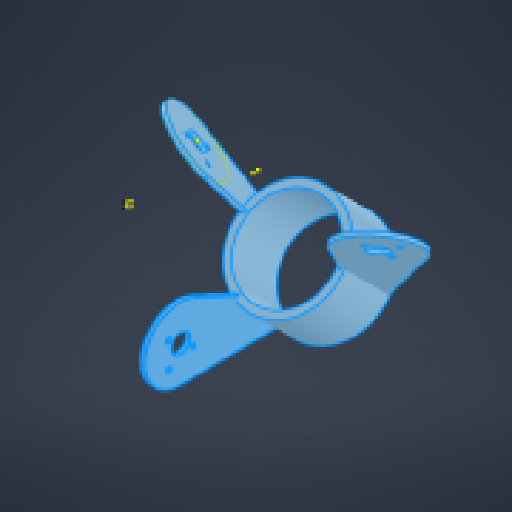
# Autodesk Inventor part: Base3MotorsHead
Saved by Autodesk Inventor 2026 (Build 300175050, 175E)
## iProperties
Created: 2025-06-26
Part Number: Base3MotorsHead
Material: Generic
Document SubType Name: Modeling
Designer: RubenPC
Density: 1 g/cm^3
Appearance: Default
Author: RubenPC
Autodesk Inventor part; units mm, degrees
ref_plane "Work Plane2" through (-10.193577, 19.428351, 24.333337) normal (0.5, 0.6123724, -0.6123724) x (-0.8659961, 0.3593609, -0.3477219)
sketch "Sketch1" plane through (-10.193577, 19.428351, 24.333337) normal (0.5, 0.6123724, -0.6123724) x (-0.8659961, 0.3593609, -0.3477219)
  circle A0 centre (-11.136116, 17.567445) radius 13.35
  circle A1 centre (-11.136116, 9.567445) radius 1.3
  circle A2 centre (-11.136116, 25.567445) radius 1.3
  circle A3 centre (-22.136116, 17.567445) radius 1.3
  circle A4 centre (-11.136116, 17.567445) radius 5
  circle A5 centre (-11.136116, 17.567445) radius 19.05
  point P0 (-7.348153, -30.884757)
  dimension "d3" = 38.1
  constraints: 1 centre point, 1 coincident
  measures "d3" diameter of A5
extrude "Extrusion1" add sketch "Sketch1" along normal blind 2 contours A0 | A5
ref_plane "Work Plane3" through (38.369556, -40.049097, 83.810785) normal (1, 0, 0) x (0, 0.8165027, -0.5773415)
ref_plane "Work Plane4" through (38.369556, -40.049097, 83.810785) normal (1, 0, 0) x (0, 0.8165027, -0.5773415)
sketch "Sketch2" plane through (38.369556, -40.049097, 83.810785) normal (1, 0, 0) x (0, 0.8165027, -0.5773415)
  circle A0 centre (14.07312, 15.315857) radius 13.35
  circle A1 centre (14.07312, 7.315857) radius 1.3
  circle A2 centre (14.07312, 23.315857) radius 1.3
  circle A3 centre (3.07312, 15.315857) radius 1.3
  circle A4 centre (14.07312, 15.315857) radius 5
  circle A5 centre (14.07312, 15.315857) radius 19.05
  point P0 (81.087646, -45.309729)
  dimension "d2" = 38.1
  constraints: 1 centre point, 1 coincident
  measures "d2" diameter of A5
extrude "Extrusion2" add sketch "Sketch2" along normal blind 2 separate body contours A0 | A5
ref_plane "Work Plane5" through (77.39899, 56.579392, 52.285482) normal (0.5, -0.6123724, 0.6123724) x (0.7923994, 0.6088063, -0.038185)
sketch "Sketch4" plane through (0.575465, 29.021734, 39.45362) normal (0.5, 0.6123724, -0.6123724) x (-0.7745967, 0, -0.6324555)
  circle A0 centre (0, 0) radius 19.05 projected
  circle A1 centre (0, 0) radius 19.05 projected
  point P0 (25.398414, -41.435313)
sketch "Sketch8" plane through (-10.193577, 19.428351, 24.333337) normal (0.5, 0.6123724, -0.6123724) x (-0.8659961, 0.3593609, -0.3477219)
  circle A0 centre (-11.136116, 17.567445) radius 19.05
  line L0 (-29.456151, 22.790356) -> (-37.949033, 0.312331)
  line L1 (-38.236466, -34.611486) -> (2.996032, 4.79306)
  line L2 (-38.236466, -34.611486) -> (-37.949033, 0.312331)
  point P0 (-7.348153, -30.884757)
  point P1 (0.984757, 2.87095)
  point P2 (-30.144601, 16.31047)
  constraints: 6 end point, 2 point on circle, 3 other
ref_plane "Work Plane7" through (48.769556, 20.910804, 22.850885) normal (0, 0.7071068, 0.7071068) x (0, 0.7071068, -0.7071068)
sketch "Sketch11" plane through (48.769556, 20.910804, 22.850885) normal (0, 0.7071068, 0.7071068) x (0, 0.7071068, -0.7071068)
  circle A0 centre (-24.13, 0) radius 24.13 projected
  circle A1 centre (-24.13, 0) radius 27.94
  point P0 (1.371844, 48.769556)
  dimension "d19" = 55.88
  constraints: 1 centre point, 1 coincident
  measures "d19" diameter of A1
extrude "Extrusion7" add sketch "Sketch11" against normal blind 33.812505 separate body
ref_plane "Work Plane8" through (97.963646, 27.796989, 40.678365) normal (-0.5, 0.6123724, -0.6123724) x (-0.8483483, -0.4884756, 0.2041979)
sketch "Sketch12" plane through (97.963646, 27.796989, 40.678365) normal (-0.5, 0.6123724, -0.6123724) x (-0.8483483, -0.4884756, 0.2041979)
  circle A0 centre (0, 0) radius 13.35 projected
  circle A1 centre (0, -8) radius 1.3 projected
  circle A2 centre (0, 8) radius 1.3 projected
  circle A3 centre (-11, 0) radius 1.3 projected
  circle A4 centre (0, 0) radius 5 projected
  circle A5 centre (0, 0) radius 19.05
  point P0 (88.379006, -31.292647)
  dimension "d24" = 38.1
  constraints: 1 centre point, 1 coincident
  measures "d24" diameter of A5
extrude "Extrusion9" add sketch "Sketch12" along normal blind 2 separate body contours A0 | A5
sketch "Sketch13" plane through (97.963646, 27.796989, 40.678365) normal (-0.5, 0.6123724, -0.6123724) x (-0.8483483, -0.4884756, 0.2041979)
  line L0 (36.658828, -45.969558) -> (29.63839, -11.757439)
  line L1 (29.63839, -11.757439) -> (14.105649, 12.803639)
  circle A0 centre (0, 0) radius 19.05
  line L2 (36.658828, -45.969558) -> (-12.394751, -14.466259)
  point P0 (88.379006, -31.292647)
  point P1 (17.61391, 7.256217)
  point P2 (-7.999269, -17.289135)
  constraints: 6 end point, 2 point on circle, 3 other
extrude "Extrusion10" add sketch "Sketch13" along normal blind 2 separate body contours L2 A0 L1 L0
extrude "Extrusion11" add sketch "Sketch8" along normal blind 2 separate body contours A0 L1 L2 L0
sketch "Sketch14" plane through (40.369556, -19.715875, 88.191228) normal (1, 0, 0) x (0, 0, -1)
  line L0 (55.911075, -18.193999) -> (31.21537, 6.501705)
  line L1 (31.21537, 6.501705) -> (6.584901, 17.875726)
  circle A0 centre (0, 0) radius 19.05
  line L2 (55.911075, -18.193999) -> (0, -19.05)
  point P0 (88.191228, 19.715875)
  point P1 (9.33763, 16.604553)
  point P2 (0.583176, -19.041072)
  constraints: 6 end point, 2 point on circle, 3 other
sketch "Sketch14 outline for Extrusion12" plane through (40.369556, -19.715875, 88.191228) normal (1, 0, 0) x (0, 0, -1)
  line L0 (55.911075, -18.193999) -> (31.21537, 6.501705)
  line L1 (0.583176, -19.041072) -> (55.911075, -18.193999)
  arc A0 (9.33763, 16.604553) -> (0.583176, -19.041072) centre (0, 0) cw
  line L2 (31.21537, 6.501705) -> (9.33763, 16.604553)
extrude "Extrusion12" add sketch "Sketch14 outline for Extrusion12" against normal blind 2 separate body
combine bodies "Aleta Inferior" operation type add bodies to combine 7 2
combine bodies "AletaSuperiorIzq" operation type add bodies to combine 1 6
combine bodies "AletaSuperiorDer" operation type add bodies to combine 5 4
body "Solid7"
body "Solid9"
body "Solid11"
